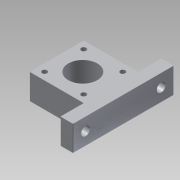
# Autodesk Inventor part: Stepper Holder X&Y
Saved by Autodesk Inventor 2014 (Build 180170000, 170)
## iProperties
Created: 2015-06-04
Part Number: Stepper Holder X&Y
Material: Aluminum 6061
Document SubType Name: Modeling
Designer: Mathias L. Kjeldgaard
Density: 2.71 g/cm^3
Appearance: Aluminum - Flat
Mass: 116.235 g
Surface Area: 123.881 cm^2
Volume: 42.8912 cm^3
Author: Mathias L. Kjeldgaard
Autodesk Inventor part; units mm, degrees
ref_plane "YZ Plane" through (0, 0, 0) normal (1, 0, 0) x (0, 1, 0)
ref_plane "XZ Plane" through (0, 0, 0) normal (0, 1, 0) x (-1, 0, 0)
ref_plane "Work Plane1" through (0, -862.1118, 0) normal (0, 0, 1) x (-1, 0, 0)
sketch "Sketch1" plane through (0, -862.1118, 0) normal (0, 0, 1) x (-1, 0, 0)
  circle A0 centre (-188, -18) radius 4 projected
  line L0 (-220, -478) -> (-220, 22) projected
  line L1 (-220, -478) -> (-208, -478) projected
  line L2 (-208, 22) -> (-208, -478) projected
  line L3 (-220, 22) -> (-208, 22) projected
  line L4 (-208, -27.0151) -> (-198, -27.0151)
  line L5 (-198, -107.0151) -> (-208, -107.0151)
  line L6 (-208, -107.0151) -> (-208, -27.0151)
  line L7 (-155, -45.5151) -> (-198, -45.5151)
  line L8 (-198, -88.5151) -> (-155, -88.5151)
  line L9 (-155, -88.5151) -> (-155, -45.5151)
  circle A1 centre (-176.15, -66.6651) radius 11.5
  circle A2 centre (-161, -51.5151) radius 2
  circle A3 centre (-192, -51.5151) radius 2
  circle A4 centre (-192, -82.5151) radius 2
  circle A5 centre (-161, -82.5151) radius 2
  line L10 (-192, -82.5151) -> (-192, -51.5151) construction
  line L11 (-192, -82.5151) -> (-161, -82.5151) construction
  line L12 (-198, -27.0151) -> (-198, -45.5151)
  line L13 (-198, -88.5151) -> (-198, -107.0151)
  point P0 (0, -862.1118)
  dimension "d0" = 10
  dimension "d1" = 80
  dimension "d3" = 43
  dimension "d4" = 18.5
  dimension "d5" = 18.5
  dimension "d6" = 23
  dimension "d7" = 4
  dimension "d8" = 4
  dimension "d9" = 4
  dimension "d10" = 4
  dimension "d11" = 31
  dimension "d12" = 31
  dimension "d13" = 31
  dimension "d14" = 31
  dimension "d15" = 6
  dimension "d18" = 6
  dimension "d19" = 6
  dimension "d20" = 6
  dimension "d21" = 90
  dimension "d25" = 21.15
  dimension "d26" = 21.15
  dimension "d27" = 90
  dimension "d28" = 90
  dimension "d29" = 18.5
  constraints: 20 end point, 5 centre point, 4 parallel, 3 perpendicular, 2 horizontal, 1 point on line
  measures "d0" distance of L5.start L5.end
  measures "d1" distance of L4.end L5.start
  measures "d3" distance between parallel lines of L8 L7
  measures "d4" distance between parallel lines of L4 L7
  measures "d5" distance between parallel lines of L5 L8
  measures "d6" diameter of A1
  measures "d7" diameter of A2
  measures "d8" diameter of A3
  measures "d9" diameter of A4
  measures "d10" diameter of A5
  measures "d11" distance of L10.end A2.centre
  measures "d12" distance of L10.start L10.end
  measures "d13" distance of L11.end L10.start
  measures "d14" distance of A2.centre L11.end
  measures "d15" distance from line of L9 A2.centre
  measures "d18" distance from line of L8 L11.end
  measures "d19" distance from line of L8 L10.start
  measures "d20" distance from line of L7 L10.end
  measures "d21" angle of L11 L10
  measures "d25" distance from line of L7 A1.centre
  measures "d26" distance from line of L9 A1.centre
  measures "d27" angle of L13 L8
  measures "d28" angle of L12 L7
  measures "d29" distance of L4.end L7.end
extrude "Tykkelse" add sketch "Sketch1" along normal blind 20 contours L2 L4 L12 L7 L9 L8 L13 L5
sketch "Sketch2" plane through (198, -835.0967, 0) normal (-1, 0, 0) x (0, 0, 1)
  line L0 (0, 0) -> (20, 0) projected
  line L1 (20, 18.5) -> (20, 0) projected
  line L2 (0, 80) -> (0, 61.5) projected
  line L3 (0, 61.5) -> (20, 61.5) projected
  line L4 (20, 80) -> (20, 61.5) projected
  line L5 (0, 80) -> (20, 80) projected
  circle A0 centre (10, 70) radius 3.5
  circle A1 centre (10, 10) radius 3.5
  point P0 (0, 835.0967)
  dimension "d32" = 7
  dimension "d33" = 7
  dimension "d34" = 10
  dimension "d35" = 10
  dimension "d36" = 10
  dimension "d37" = 10
  constraints: 2 centre point
  measures "d32" diameter of A1
  measures "d33" diameter of A0
  measures "d34" distance from line of L5 A0.centre
  measures "d35" distance from line of L4 A0.centre
  measures "d36" distance from line of L1 A1.centre
  measures "d37" distance from line of L0 A1.centre
extrude "Extrusion2" cut sketch "Sketch2" against normal up to surface (10 mm away) contours A0 | A1
fillet "Fillet1" radius 0.5 8 edges at (198, -816.5967, 10) (198, -773.5967, 10) (155, -773.5967, 10) (155, -816.5967, 10) (198, -835.0967, 10) (208, -835.0967, 10) (198, -755.0967, 10) (208, -755.0967, 10)
equation "\"d4\" = d5"
equation "\"d8\" = d7"
equation "\"d9\" = d7"
equation "\"d10\" = d7"
equation "\"d13\" = d11"
equation "\"d14\" = d12"
equation "\"d15\" = d20"
equation "\"d18\" = d15"
equation "\"d19\" = d18"
body "Solid1"
